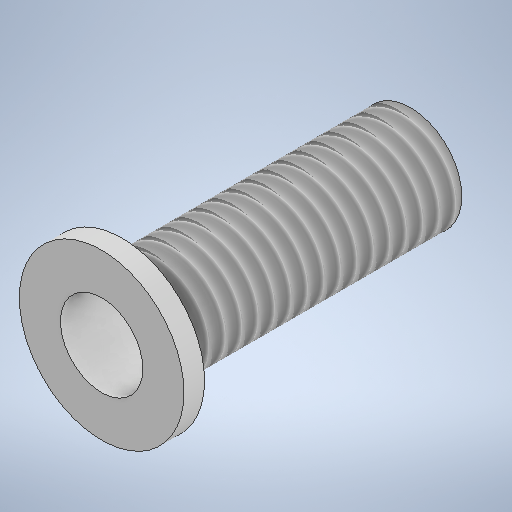
# Autodesk Inventor part: Resistencia_Tornillo
Saved by Autodesk Inventor 2026 (Build 300175050, 175E)
## iProperties
Created: 2025-05-26
Part Number: Resistencia_Tornillo
Material: Genérico
Document SubType Name: Modeling
Designer: alex
Density: 1 g/cm^3
Appearance: Valor por defecto
Author: alex
Autodesk Inventor part; units mm, degrees
ref_plane "YZ Plane" through (0, 0, 0) normal (1, 0, 0) x (0, 1, 0)
ref_plane "XZ Plane" through (0, 0, 0) normal (0, 1, 0) x (-1, 0, 0)
ref_plane "XY Plane" through (0, 0, 0) normal (0, 0, 1) x (1, 0, 0)
sketch "Boceto1" plane through (0, 0, 0) normal (0, 0, 1) x (1, 0, 0)
  circle A0 centre (0, 0) radius 2
  circle A1 centre (0, 0) radius 2.5
  dimension "d0" = 4
  dimension "d1" = 5
  constraints: 2 centre point, 2 coincident
  measures "d0" diameter of A0
  measures "d1" diameter of A1
extrude "Extrusión1" add sketch "Boceto1" against normal blind 15
sketch "Boceto2" plane through (0, 0, 0) normal (0, 0, 1) x (1, 0, 0)
  circle A0 centre (0, 0) radius 2.5 projected
  circle A1 centre (0, 0) radius 4
  circle A2 centre (0, 0) radius 2.5
  dimension "d5" = 8
  constraints: 2 centre point, 2 coincident, 1 concentric
  measures "d5" diameter of A1
extrude "Extrusión2" add sketch "Boceto2" against normal blind 1
thread "Rosca1" size "M5x0.8" class "6g" standard "ANSI Metric M Profile" full length
